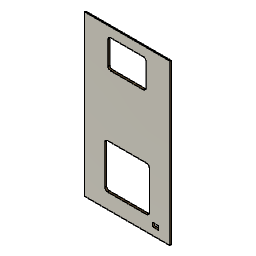
back_panel (Autodesk Fusion 360 design; units mm, degrees)
Autodesk Fusion 360 part; units mm, degrees
sketch "Back Panel" plane through (0, 0, 0) normal (1, 0, 0) x (0, 1, 0)
  line L0 (0, 0) -> (6, 0)
  line L1 (6, 0) -> (6, 500.8)
  line L2 (0, 500.8) -> (0, 0)
  line L3 (0, 500.8) -> (0, 503.263)
  line L4 (6, 500.8) -> (0, 503.263)
  dimension "d8" = 6
  dimension "d9" = 500.8
  dimension "d10" = 2.463
  dimension "d11" = 112.318
  constraint horizontal L0
  constraint vertical L1
  constraint vertical L2
  constraint coincident L0.start L2.end
  measures "d8" distance of L0.start L0.end
  measures "d9" distance of L0.end L1.end
  measures "d10" distance of L2.start L3.end
  measures "d11" angle of L1 L4
extrude "Extrude2" add sketch "Back Panel" along normal blind 270
sketch "Switch Hole" plane through (0, 6, 0) normal (0, 1, 0) x (-1, 0, 0)
  line L0 (0, 0) -> (0, 500.8)
  line L1 (0, 500.8) -> (-270, 500.8)
  line L2 (-270, 500.8) -> (-270, 0)
  line L3 (-270, 0) -> (0, 0)
  line L4 (-234, 36) -> (-216, 36)
  line L5 (-216, 36) -> (-216, 24)
  line L6 (-216, 24) -> (-234, 24)
  line L7 (-234, 24) -> (-234, 36)
  dimension "d14" = 18
  dimension "d15" = 12
  dimension "d16" = 36
  dimension "d17" = 24
  constraint horizontal L4
  constraint vertical L5
  constraint horizontal L6
  constraint vertical L7
  measures "d14" distance of L5.end L6.end
  measures "d15" distance of L4.end L5.end
  measures "d16" distance of L2 L7
  measures "d17" distance of L3 L6
extrude "Extrude3" cut sketch "Switch Hole" against normal blind 6 contours L4 L5 L6 L7
sketch "Bottom Access Panel" plane through (0, 6, 0) normal (0, 1, 0) x (-1, 0, 0)
  line L0 (-216, 36) -> (-216, 24)
  line L1 (-216, 24) -> (-234, 24)
  line L2 (-234, 24) -> (-234, 36)
  line L3 (-234, 36) -> (-216, 36)
  line L4 (0, 0) -> (0, 500.8)
  line L5 (0, 500.8) -> (-270, 500.8)
  line L6 (-270, 500.8) -> (-270, 0)
  line L7 (-270, 0) -> (0, 0)
  line L8 (-205, 188) -> (-65, 188)
  line L9 (-65, 188) -> (-65, 48)
  line L10 (-65, 48) -> (-205, 48)
  line L11 (-205, 48) -> (-205, 188)
  dimension "d20" = 48
  dimension "d21" = 65
  dimension "d22" = 65
  dimension "d28" = 140
  dimension "d29" = 140
  dimension "d30" = 24
  dimension "d31" = 12
  dimension "d32" = 12
  dimension "d33" = 188
  constraint horizontal L8
  constraint vertical L9
  constraint horizontal L10
  constraint vertical L11
  measures "d20" distance of L7 L10
  measures "d21" distance of L6 L11
  measures "d22" distance of L4 L9
  measures "d28" distance of L8.end L9.end
  measures "d29" distance of L9.end L10.end
  measures "d30" distance of L1 L7
  measures "d31" distance of L3 L10
  measures "d32" distance of L1 L3
  measures "d33" distance of L7 L8
extrude "Extrude4" cut sketch "Bottom Access Panel" against normal blind 6 contours L8 L9 L10 L11
fillet "Fillet1" radius 8 4 edges at (65, 3, 188) (65, 3, 48) (205, 3, 48) (205, 3, 188)
sketch "Top Access Panel" plane through (0, 6, 0) normal (0, 1, 0) x (-1, 0, 0)
  line L0 (-65, 180) -> (-65, 56)
  arc A0 (-73, 48) -> (-65, 56) centre (-73, 56) ccw
  line L1 (-73, 48) -> (-197, 48)
  arc A1 (-205, 56) -> (-197, 48) centre (-197, 56) ccw
  line L2 (-205, 56) -> (-205, 180)
  arc A2 (-197, 188) -> (-205, 180) centre (-197, 180) ccw
  line L3 (-197, 188) -> (-73, 188)
  arc A3 (-65, 180) -> (-73, 188) centre (-73, 180) ccw
  line L4 (-216, 36) -> (-216, 24)
  line L5 (-216, 24) -> (-234, 24)
  line L6 (-234, 24) -> (-234, 36)
  line L7 (-234, 36) -> (-216, 36)
  line L8 (0, 0) -> (0, 500.8)
  line L9 (0, 500.8) -> (-270, 500.8)
  line L10 (-270, 500.8) -> (-270, 0)
  line L11 (-270, 0) -> (0, 0)
  line L12 (-195, 473.263) -> (-75, 473.263)
  line L13 (-75, 473.263) -> (-75, 383.263)
  line L14 (-75, 383.263) -> (-195, 383.263)
  line L15 (-195, 383.263) -> (-195, 473.263)
  line L16 (-180, 473.263) -> (-90, 473.263)
  line L17 (0, 503.263) -> (-270, 503.263)
  dimension "d34" = 120
  dimension "d35" = 140
  dimension "d36" = 75
  dimension "d37" = 75
  dimension "d38" = 65
  dimension "d39" = 65
  dimension "d45" = 90
  dimension "d49" = 30
  constraint horizontal L12
  constraint vertical L13
  constraint horizontal L14
  constraint vertical L15
  constraint coincident L12 L16.start
  measures "d34" distance of L13.end L14.end
  measures "d35" distance of L0 L2
  measures "d36" distance of L10 L15
  measures "d37" distance of L8 L13
  measures "d38" distance of L2 L10
  measures "d39" distance of L0 L8
  measures "d45" distance of L12.end L13.end
  measures "d49" distance of L16 L17
extrude "Extrude5" cut sketch "Top Access Panel" against normal blind 6 contours L12 L13 L14 L15 L16
fillet "Fillet2" radius 8 4 edges at (75, 3, 473.263) (195, 3, 473.263) (195, 3, 383.263) (75, 3, 383.263)
equation "MDFThickness = 6 mm" comment "Thickness of the MDF board"
equation "d16 = ( 18 * 2 ) * 1 mm"
equation "d17 = ( 12 * 2 ) * 1 mm"
equation "d18 = -MDFThickness"
equation "d23 = -MDFThickness"
equation "filletRadius = 8 mm" comment "Radius to use for fillets"
equation "d27 = filletRadius"
equation "d36 = ( ( 270 - 120 ) / 2 ) * 1 mm"
equation "d51 = -MDFThickness"
equation "d54 = filletRadius"
named bodies: "Back Panel"
